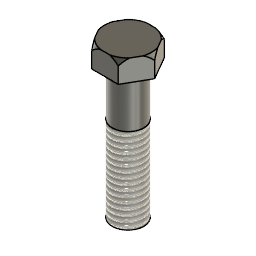
Screw (Autodesk Fusion 360 design; units mm, degrees)
Autodesk Fusion 360 part; units mm, degrees
sketch "Sketch1" plane through (0, 0, 0) normal (0, 0, 1) x (1, 0, 0)
  circle A0 centre (0, 0) radius 4.7625
  dimension "d1" = 9.525
  constraint coincident A0.centre origin
  measures "d1" diameter of A0
extrude "Extrude1" add sketch "Sketch1" along normal blind 25.4 makes body 1
thread "Thread1" "ANSI Unified Screw Threads 0.375 3/8-16 UNC 3/8-16 UNC 3A" major diameter 9.4056 minor diameter 7.6327 pitch 1.5875 angle 60 resizes the face on face at (4.7388, -0.4742, 16.9333) on bodies 1
sketch "Sketch2" plane through (0, 0, 25.4) normal (0, 0, 1) x (-1, 0, 0)
  circle A0 centre (0, 0) radius 4.7028
  circle A1 centre (0, 0) radius 4.7625
  dimension "d6" = 9.525
  constraint coincident A0.centre A1.centre
  measures "d6" diameter of A1
extrude "Extrude2" add sketch "Sketch2" along normal blind 14.2875 separate body contours A0 makes body 2
sketch "Sketch3" plane through (0, 0, 39.6875) normal (0, 0, 1) x (-1, 0, 0)
  circle A0 centre (0, 0) radius 4.7028
  circle A1 centre (0, 0) radius 7.9375
  line L0 (-7.9375, 0) -> (-3.9688, -6.8741)
  line L1 (-3.9688, -6.8741) -> (3.9687, -6.8741)
  line L2 (3.9687, -6.8741) -> (7.9375, 0)
  line L3 (7.9375, 0) -> (3.9688, 6.8741)
  line L4 (3.9688, 6.8741) -> (-3.9687, 6.8741)
  line L5 (-3.9687, 6.8741) -> (-7.9375, 0)
  dimension "d9" = 15.875
  constraint coincident A0.centre A1.centre
  constraint coincident A1 L0.start
  measures "d9" diameter of A1
extrude "Extrude3" add sketch "Sketch3" along normal blind 6.35 contours A0 | L0 L1 L2 L3 L4 L5 bodies 2
sketch "Sketch4" plane through (0, 0, 0) normal (0, 1, 0) x (1, 0, 0)
  line L0 (-7.021, -39.6875) -> (-7.9375, -41.275)
  line L1 (-7.9375, -39.6875) -> (-7.9375, -46.0375)
  line L2 (-7.9375, -39.6875) -> (-3.9688, -39.6875)
  line L3 (-7.021, -46.0375) -> (-7.9375, -44.45)
  line L4 (-7.9375, -46.0375) -> (-3.9688, -46.0375)
  line L5 (-7.9375, -46.0375) -> (-7.021, -46.0375)
  line L6 (-7.9375, -46.0375) -> (-7.9375, -44.45)
  line L7 (-7.9375, -39.6875) -> (-7.9375, -41.275)
  line L8 (-7.9375, -39.6875) -> (-7.021, -39.6875)
  dimension "d12" = 1.5875
  dimension "d13" = 150
  dimension "d14" = 1.5875
  dimension "d15" = 150
  constraint coincident L0.end L1
  constraint coincident L0.start L2
  constraint coincident L3.start L4
  constraint coincident L1 L3.end
  constraint coincident L1.end L4.start
  constraint coincident L1.start L2.start
  measures "d12" distance of L0.end L1.start
  measures "d13" angle of L0 L1
  measures "d14" distance of L1.end L3.end
  measures "d15" angle of L1 L3
revolve "Revolve1" cut sketch "Sketch4" angle 360 about axis through (0, 0, 25.4) along (0, 0, -1) contours L1 L3 L4 L5 L6 bodies 2
equation "d9 = ( 5 / 8 ) * 1 in"
